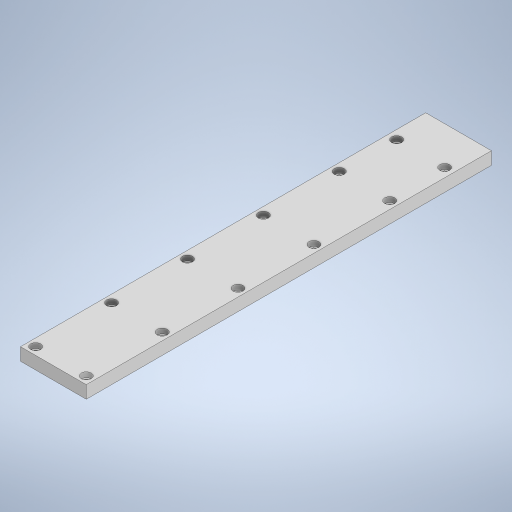
# Autodesk Inventor part: body_cover_v2
Saved by Autodesk Inventor 2023 (Build 270158000, 158)
## iProperties
Created: 2023-07-18
Part Number: body_cover_v2
Material: Generic
Document SubType Name: Modeling
Designer: checo
Density: 1 g/cm^3
Appearance: Default
Author: checo
Autodesk Inventor part; units mm, degrees
ref_plane "YZ Plane" through (0, 0, 0) normal (1, 0, 0) x (0, 1, 0)
ref_plane "XZ Plane" through (0, 0, 0) normal (0, 1, 0) x (-1, 0, 0)
ref_plane "XY Plane" through (0, 0, 0) normal (0, 0, 1) x (1, 0, 0)
sketch "Sketch1" plane through (0, 0, 0) normal (0, 1, 0) x (-1, 0, 0)
  line L0 (-13, -80.1) -> (13, -80.1)
  line L1 (13, -80.1) -> (13, 80.1)
  line L2 (13, 80.1) -> (-13, 80.1)
  line L3 (-13, 80.1) -> (-13, -80.1)
  line L4 (-13, -80.1) -> (13, 80.1) construction
  line L5 (13, -80.1) -> (-13, 80.1) construction
  point P0 (0, 0)
  dimension "d0" = 160.2
  dimension "d1" = 26
  constraints: 12 end point, 2 midpoint, 2 parallel, 1 horizontal, 1 perpendicular
  measures "d0" distance of L0.end L1.end
  measures "d1" distance of L1.end L2.end
extrude "Extrusion1" add sketch "Sketch1" along normal blind 5
sketch "Sketch2" plane through (0, 5, 0) normal (0, 1, 0) x (1, 0, 0)
  line L0 (-13, 80.1) -> (-13, -80.1) projected
  line L1 (-13, -80.1) -> (13, -80.1) projected
  line L2 (0, -80.1) -> (0, 80.1) construction
  line L3 (13, 80.1) -> (-13, 80.1) projected
  point P0 (0, 0)
  point P1 (-10, -77.1)
  point P2 (-10, -47.1)
  point P3 (-10, -17.1)
  point P4 (-10, 12.9)
  point P5 (-10, 42.9)
  point P6 (-9.5, 65.1)
  point P7 (10, -77.1)
  point P8 (10, -47.1)
  point P9 (10, -17.1)
  point P10 (10, 12.9)
  point P11 (10, 42.9)
  point P12 (9.5, 65.1)
  dimension "d4" = 3
  dimension "d5" = 3
  dimension "d8" = 30
  dimension "d13" = 15
  constraints: 6 symmetric about line, 2 end point, 2 midpoint, 1 vertical, 4 other
  measures "d4" distance from line of point (-10, -77.1) L0
  measures "d5" distance from line of point (-10, -77.1) L1
  measures "d8" distance of point (-10, -77.1) point (-10, -47.1)
  measures "d13" distance from line of L3 point (-9.5, 65.1)
hole "Hole1" at (-10, 5, 77.1) at (-10, 5, 47.1) at (-10, 5, 17.1) at (-10, 5, -12.9) at (-10, 5, -42.9) at (-9.5, 5, -65.1) at (10, 5, 77.1) at (10, 5, 47.1) at (10, 5, 17.1) at (10, 5, -12.9) at (10, 5, -42.9) at (9.5, 5, -65.1) direction (0, -1, 0) diameter 2.3813 depth 10 tip angle 118 counterbore diameter 4 counterbore depth 2
sketch "Sketch3" plane through (13, 0, -80.1) normal (0, 0, -1) x (-1, 0, 0)
  line L0 (0, 0) -> (0, 5) projected
  line L1 (0, 2.5) -> (26, 2.5) construction
  line L2 (26, 0) -> (26, 5) projected
  line L3 (26, 5) -> (0, 5) construction
  line L4 (13, 5) -> (13, 0) construction
  line L5 (26, 0) -> (0, 0) construction
  point P0 (3, 2.5)
  point P1 (23, 2.5)
  dimension "d22" = 3
  constraints: 4 end point, 3 midpoint, 1 perpendicular, 1 point on line, 1 symmetric about line
  measures "d22" distance from line of L0 point (3, 2.5)
hole "Hole2" at (10, 2.5, -80.1) at (-10, 2.5, -80.1) direction (0, 0, 1) diameter 2.3813 depth 10 tip angle 118
sketch "Sketch4" plane through (0, 0, 0) normal (0, -1, 0) x (1, 0, 0)
  line L0 (13, 80.1) -> (13, -80.1) projected
  line L1 (-13, 80.1) -> (13, 80.1) projected
  line L2 (-13, -80.1) -> (-13, 80.1) projected
  line L3 (13, -80.1) -> (-13, -80.1) projected
  line L4 (10, -77.1) -> (10, 77.1) construction
  line L5 (10, 77.1) -> (-10, 77.1) construction
  line L6 (-10, 77.1) -> (-10, -77.1) construction
  line L7 (-10, -77.1) -> (10, -77.1) construction
  point P0 (0, 0)
  dimension "d30" = 3
  constraints: 8 end point, 3 other
  measures "d30" distance between parallel lines of L0 L4
sketch "Sketch5" plane through (-13, 0, 80.1) normal (0, 0, 1) x (1, 0, 0)
  line L0 (0, 0) -> (26, 0) projected
  circle A0 centre (23, 0) radius 0.25
  point P0 (13, 0)
  point P1 (23.25, 0)
  point P2 (22.75, 0)
  dimension "d31" = 3
  dimension "d32" = 0.5
  constraints: 1 centre point, 1 point on line
  measures "d31" distance of L0.end A0.centre
  measures "d32" diameter of A0
sweep "Sweep1" cut profiles "Sketch5" path "Sketch4" picked at (23.0624, 0.0951) path curves L0 L3 L2 L1 contours A0 L0
body "Solid1"
